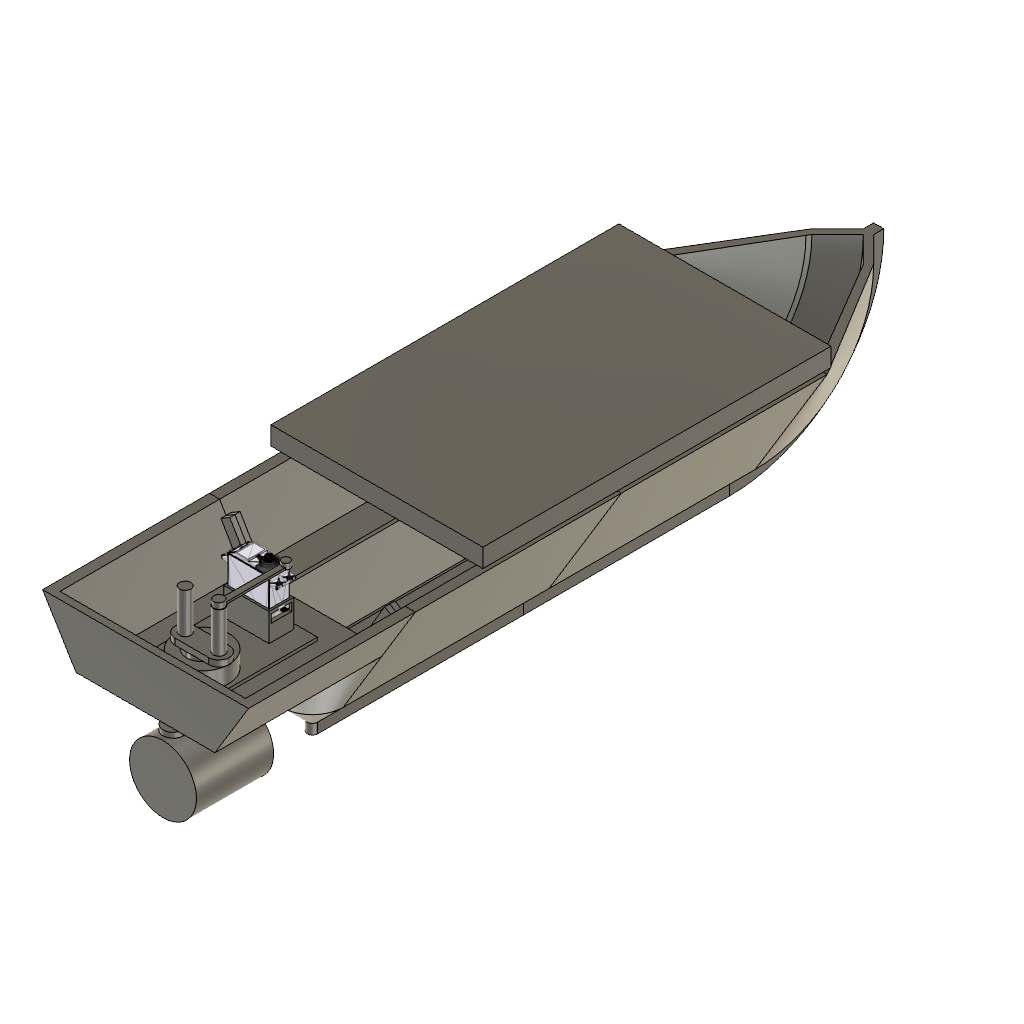
Aleph 0.2 (Autodesk Fusion 360 design; units mm, degrees)
part number: 2025-10-31-18-29-23-563
Autodesk Fusion 360 part; units mm, degrees
note: some values were not read from the file. Chosen so that the rebuilt part matches the saved one: a direction; which face or edge a step refers to. Set by a fixed rule: which sketch regions a step uses.
sketch "Skizze2" plane through (0, 0, 0) normal (0, 0, 1) x (1, 0, 0)
  line L0 (0, 0) -> (43, 0)
  line L1 (43, 0) -> (43, -97)
  line L2 (43, -97) -> (0, -97)
  line L3 (0, -97) -> (0, 0)
  dimension "d1" = 43
  dimension "d2" = 97
  constraint horizontal L0
  constraint vertical L1
  constraint horizontal L2
  constraint vertical L3
  constraint coincident L0.start L3.end
  measures "d1" distance of L0.start L0.end
  measures "d2" distance of L0.start L2.end
extrude "Extrusion1" add sketch "Skizze2" along normal blind 52 makes body 1
sketch "Skizze4" plane through (0, 0, 0) normal (0, 0, 1) x (1, 0, 0)
  line L0 (0, 0) -> (114.3, 0)
  line L1 (114.3, 0) -> (114.3, -187.452)
  line L2 (114.3, -187.452) -> (0, -187.452)
  line L3 (0, -187.452) -> (0, 0)
  dimension "d5" = 114.3
  dimension "d6" = 187.452
  constraint horizontal L0
  constraint vertical L1
  constraint horizontal L2
  constraint vertical L3
  constraint coincident L0.start L3.end
  measures "d5" distance of L0.start L0.end
  measures "d6" distance of L0.start L2.end
extrude "Extrusion2" add sketch "Skizze4" along normal blind 44.45 separate body makes body 2
move_body "Verschieben1" bodies 1 to x (0, -1, 0) y (1, 0, 0) z (0, 0, 1) at (47, -192, 0)
move_body "Verschieben2" bodies 2 to x (1, 0, 0) y (0, 1, 0) z (0, 0, 1) at (-60, 0, 0)
sketch "Skizze5" plane through (0, 0, 0) normal (0, 0, 1) x (1, 0, 0)
  line L0 (0, 0) -> (-57, 0)
  line L1 (-57, 0) -> (-57, 115)
  line L2 (-57, 115) -> (0, 115)
  line L3 (0, 115) -> (0, 0)
  dimension "d9" = 57
  dimension "d10" = 115
  constraint horizontal L0
  constraint vertical L1
  constraint horizontal L2
  constraint vertical L3
  constraint coincident L0.start L3.end
  measures "d9" distance of L0.start L0.end
  measures "d10" distance of L0.start L2.end
extrude "Extrusion3" add sketch "Skizze5" along normal blind 20 separate body makes body 3
move_body "Verschieben3" bodies 3 to x (-1, 0, 0) y (0, -1, 0) z (0, 0, 1) at (-32.12, -30.0306, 0.3149)
sketch "Skizze6" plane through (0, 0, 0) normal (0, 0, 1) x (1, 0, 0)
  line L0 (0, 0) -> (-340, 0)
  line L1 (-340, 0) -> (-340, 190)
  line L2 (-340, 190) -> (0, 190)
  line L3 (0, 190) -> (0, 0)
  dimension "d13" = 340
  dimension "d14" = 190
  constraint horizontal L0
  constraint vertical L1
  constraint horizontal L2
  constraint vertical L3
  constraint coincident L0.start L3.end
  measures "d13" distance of L0.start L0.end
  measures "d14" distance of L0.start L2.end
move_body "Verschieben5" bodies 1 to x (0, 1, 0) y (-1, 0, 0) z (0, 0, 1) at (-215.4447, -91.9643, -60)
sketch "Skizze8" plane through (0, 0, 19.9339) normal (0, 0, 1) x (-1, 0, 0)
  line L0 (-89.3962, 276.7581) -> (-89.3962, -63.2419)
  line L1 (-89.3962, -63.2419) -> (100.6038, -63.2419)
  line L2 (100.6038, -63.2419) -> (100.6038, 276.7581)
  line L3 (100.6038, 276.7581) -> (-89.3962, 276.7581)
  line L4 (0, 0) -> (206, 0)
  line L5 (206, 0) -> (206, -338)
  line L6 (206, -338) -> (0, -338)
  line L7 (0, -338) -> (0, 0)
  dimension "d17" = 206
  dimension "d18" = 338
  constraint horizontal L4
  constraint vertical L5
  constraint horizontal L6
  constraint vertical L7
  constraint coincident L4.start L7.end
  measures "d17" distance of L4.start L4.end
  measures "d18" distance of L4.start L6.end
extrude "Extrusion5" add sketch "Skizze8" along normal blind 18 separate body contours L1 L2 L4 L7 | L1 L2 L4 L5 L6 L7 makes body 4
move_body "Verschieben7" bodies 4 to x (1, 0, 0) y (0, 1, 0) z (0, 0, 1) at (95.4562, -274.0751, 0)
move_body "Verschieben8" bodies 4 to x (1, 0, 0) y (0, 1, 0) z (0, 0, 1) at (2.397, 0, -6.8914)
sketch "Skizze9" plane through (0, 0, 0) normal (0, 1, 0) x (1, 0, 0)
  line L0 (5, 140) -> (-5, 140)
  line L1 (-5, 140) -> (-30, 115)
  line L2 (29.8931, 115.1069) -> (5, 140)
  line L3 (-25, 110) -> (0, 135)
  line L4 (0, 135) -> (25, 110)
  line L5 (-25, 110) -> (-15, 110)
  line L6 (-15, 110) -> (-15, 106.5)
  line L7 (-15, 106.5) -> (-27.2273, 106.5)
  line L8 (5, 140) -> (5, 150)
  line L9 (5, 150) -> (-5, 150)
  line L10 (-5, 150) -> (-5, 140)
  line L11 (25, 110) -> (15, 110)
  line L12 (15, 110) -> (15, 106.5)
  line L13 (15, 106.5) -> (27.0682, 106.5)
  line L14 (-60.5574, 49.9522) -> (-35, 49.9522)
  line L15 (-35, 49.9522) -> (-35, 46.4522)
  line L16 (-35, 46.4522) -> (-62.6204, 46.4522)
  line L17 (60.4828, 49.9522) -> (35, 49.9522)
  line L18 (35, 49.9522) -> (35, 46.4522)
  line L19 (35, 46.4522) -> (62.551, 46.4522)
  line L20 (-90, 0) -> (-27.2273, 106.5)
  line L21 (-100, 0) -> (-30, 115)
  line L22 (90, 0) -> (27.0682, 106.5)
  line L23 (29.8931, 115.1069) -> (100, 0)
  line L24 (100, 0) -> (90, 0)
  line L25 (25, 110) -> (27.0682, 106.5)
  line L26 (-27.2273, 106.5) -> (-25, 110)
  line L27 (-100, 0) -> (-90, 0)
  line L28 (83.7574, 10.5643) -> (75.1482, 5.477)
  line L29 (75.1482, 5.477) -> (59.8863, 31.3048)
  line L30 (59.8863, 31.3048) -> (68.4956, 36.3921)
  line L31 (-68.5499, 36.3921) -> (-59.935, 31.3144)
  line L32 (-59.935, 31.3144) -> (-75.1683, 5.4697)
  line L33 (-75.1683, 5.4697) -> (-83.7832, 10.5474)
  line L34 (53.6547, 61.5074) -> (45.0455, 56.4201)
  line L35 (45.0455, 56.4201) -> (24.6963, 90.8572)
  line L36 (24.6963, 90.8572) -> (33.3055, 95.9445)
  line L37 (-33.4489, 95.9445) -> (-24.834, 90.8667)
  line L38 (-24.834, 90.8667) -> (-45.145, 56.4071)
  line L39 (-45.145, 56.4071) -> (-53.7599, 61.4849)
  line L40 (10, 125) -> (-10, 125)
  line L41 (71.7079, 46.4522) -> (-71.7247, 46.4522)
  line L42 (67.4445, 53.4522) -> (-67.4639, 53.4522)
  line L43 (0, 135) -> (0, 150)
  line L44 (90, 0) -> (-90, 0)
  dimension "d21" = 3.5
  dimension "d23" = 3.5
  dimension "d24" = 3.5
  dimension "d35" = 10
  dimension "d36" = 30
  dimension "d37" = 10
  dimension "d38" = 30
  dimension "d39" = 10
  dimension "d40" = 40
  dimension "d41" = 10
  dimension "d42" = 40
  constraint coincident L16.end L20
  constraint horizontal L16
  constraint coincident L14.start L20
  constraint horizontal L14
  constraint coincident L17.start L22
  constraint horizontal L17
  constraint coincident L19.end L22
  constraint horizontal L19
  constraint parallel L22 L25
  constraint horizontal L27
  constraint coincident L22 L28.start
  constraint perpendicular L22 L28
  constraint perpendicular L28 L29
  constraint coincident L22 L30.end
  constraint perpendicular L22 L30
  constraint coincident L20 L31.start
  constraint perpendicular L20 L31
  constraint perpendicular L31 L32
  constraint coincident L20 L33.end
  constraint perpendicular L20 L33
  constraint coincident L22 L34.start
  constraint perpendicular L22 L34
  constraint perpendicular L34 L35
  constraint coincident L22 L36.end
  constraint perpendicular L22 L36
  constraint coincident L20 L37.start
  constraint perpendicular L20 L37
  constraint perpendicular L37 L38
  constraint coincident L20 L39.end
  constraint perpendicular L20 L39
  constraint coincident L4 L40.start
  constraint coincident L3 L40.end
  constraint parallel L11 L40
  constraint coincident L23 L41.start
  constraint coincident L21 L41.end
  constraint parallel L19 L41
  constraint coincident L23 L42.start
  constraint coincident L21 L42.end
  constraint horizontal L42
  constraint midpoint L9 L43.end
  constraint perpendicular L9 L43
  constraint parallel L27 L44
  measures "d21" distance of L5.end L6.end
  measures "d23" distance of L11.end L12.end
  measures "d24" distance of L14.end L15.end
  measures "d35" distance of L28.start L28.end
  measures "d36" distance of L28.end L29.end
  measures "d37" distance of L31.start L31.end
  measures "d38" distance of L31.end L32.end
  measures "d39" distance of L34.start L34.end
  measures "d40" distance of L34.end L35.end
  measures "d41" distance of L37.end L37.start
  measures "d42" distance of L37.end L38.end
move_body "Verschieben9" bodies 2 to x (1, 0, 0) y (0, 1, 0) z (0, 0, 1) at (0, 0, 1.39)
move_body "Verschieben10" bodies 3 to x (1, 0, 0) y (0, 1, 0) z (0, 0, 1) at (0, 0, 5)
move_body "Verschieben11" bodies 1 to x (1, 0, 0) y (0, 1, 0) z (0, 0, 1) at (0, 0, 1.5638)
move_body "Verschieben12" bodies 4 to x (1, 0, 0) y (0, 1, 0) z (0, 0, 1) at (0, -63.155, 0.694)
sketch "Skizze11" plane through (0, 0, 0) normal (0, 1, 0) x (1, 0, 0)
  circle A0 centre (0, -70) radius 32.5
  dimension "d32" = 65
  measures "d32" diameter of A0
move_body "Verschieben16" bodies 4 to x (1, 0, 0) y (0, 1, 0) z (0, 0, 1) at (5.0085, 0, -7.0491)
extrude "Extrusion10" add sketch "Skizze9" against normal blind 200 separate body contours L0 L2 L4 L22 L23 L25 L42 L43 | L0 L1 L3 L20 L21 L26 L42 L43 | L22 L23 L41 L42 | L22 L23 L24 L41 | L20 L21 L41 L42 | L20 L21 L27 L41 makes body 5
move_body "Verschieben17" bodies 2 1 to x (1, 0, 0) y (0, 1, 0) z (0, 0, 1) at (0, -5, 0)
extrude "Extrusion11" add sketch "Skizze9" against normal blind 200 contours L5 L6 L7 L26 | L11 L12 L13 L25 | L17 L18 L19 L22 L41 | L14 L15 L16 L20 L41 bodies 5
extrude "Extrusion12" add sketch "Skizze9" against normal blind 200 contours L0 L8 L9 L43 | L0 L9 L10 L43 bodies 5
extrude "Extrusion13" add sketch "Skizze9" against normal blind 5 contours L3 L4 L40 | L22 L34 L35 L36 | L22 L28 L29 L30 | L20 L37 L38 L39 | L20 L31 L32 L33 bodies 5
extrude "Extrusion14" add sketch "Skizze9" along normal blind 5 from surface at -200 contours L3 L4 L40 | L22 L34 L35 L36 | L22 L28 L29 L30 | L20 L37 L38 L39 | L20 L31 L32 L33 bodies 5
revolve "Drehen2" add sketch "Skizze9" angle 90 about axis through (1.75, 0, 0) along (1, 0, 0) separate body contours L0 L2 L4 L22 L23 L25 L42 L43 | L0 L8 L9 L43 | L0 L1 L3 L20 L21 L26 L42 L43 | L0 L9 L10 L43 | L22 L23 L41 L42 | L22 L23 L24 L41 | L20 L21 L41 L42 | L20 L21 L27 L41 makes body 6
extrude "Extrusion15" add sketch "Skizze9" along normal blind 5 contours L3 L4 L40 | L22 L34 L35 L36 | L22 L28 L29 L30 | L20 L37 L38 L39 | L20 L31 L32 L33 bodies 6
copy_body "Körper kopieren/einfügen1" bodies 5 makes body 7
move_body "Verschieben18" bodies 7 to x (1, 0, 0) y (0, 1, 0) z (0, 0, 1) at (0, -200, 0)
sketch "Skizze12" plane through (0, 0, 0) normal (0, 0, 1) x (1, 0, 0)
  line L0 (-32.5, 0) -> (-32.5, -75)
  line L1 (-32.5, -75) -> (32.5, -75)
  line L2 (32.5, -75) -> (32.5, 0)
  line L3 (32.5, 0) -> (-32.5, 0)
  circle A0 centre (0, -17.2765) radius 1.15
  circle A1 centre (0, -37.2765) radius 1.15
  circle A2 centre (0, -57.2765) radius 1.15
  line L4 (3.25, -57.2765) -> (3.25, -17)
  line L5 (-3.25, -57.2765) -> (-3.25, -17.2765)
  arc A3 (3.25, -17) -> (-3.25, -17.2765) centre (0.0059, -17.2765) ccw
  arc A4 (-3.25, -57.2765) -> (3.25, -57.2765) centre (0, -57.2765) ccw
  dimension "d59" = 75
  dimension "d60" = 65
  dimension "d61" = 2.3
  dimension "d62" = 20
  dimension "d63" = 2.3
  dimension "d64" = 20
  dimension "d65" = 2.3
  constraint perpendicular L0 L1
  constraint perpendicular L1 L2
  constraint perpendicular L0 L3
  constraint vertical L4
  constraint vertical L5
  constraint tangent L5 A3
  constraint tangent L4 A4
  constraint tangent L5 A4
  measures "d59" distance of L0.start L0.end
  measures "d60" distance of L0.end L1.end
  measures "d61" diameter of A0
  measures "d62" distance of A0.centre A1.centre
  measures "d63" diameter of A1
  measures "d64" distance of A1.centre A2.centre
  measures "d65" diameter of A2
extrude "Extrusion16" add sketch "Skizze11" against normal blind 75 separate body makes body 8
extrude "Extrusion17" add sketch "Skizze12" along normal blind 4 from surface at 102.5 contours L4 L5 A3 A4 bodies 8
move_body "Verschieben19" bodies 8 to x (1, 0, 0) y (0, 1, 0) z (0, 0, 1) at (0, -436.8438, -182.9817)
other "Grundnetzelement1"
move_body "Verschieben20" bodies 8 to x (1, 0, 0) y (0, 1, 0) z (0, 0, 1) at (0, 0, 20)
other "Ändern1"
move_body "Verschieben21" bodies 8 to x (1, 0, 0) y (0, 1, 0) z (0, 0, 1) at (0, -25, 0)
other "Ändern2"
other "Netzreparatur1"
move_body "Verschieben22" bodies 8 to x (1, 0, 0) y (0, 1, 0) z (0, 0, 1) at (0, -30, 0)
other "Ändern3"
move_body "Verschieben23" bodies 8 to x (1, 0, 0) y (0, 1, 0) z (0, 0, 1) at (0, 31.8147, -24.8688)
other "Ändern4"
extrude "Extrusion18" add sketch "Skizze9" against normal blind 130 from surface at -400 separate body contours L22 L23 L41 L42 | L22 L23 L24 L41 | L14 L15 L17 L18 L20 L22 L41 L42 | L20 L21 L41 L42 | L17 L18 L19 L22 L41 | L20 L21 L27 L41 | L14 L15 L16 L20 L41 makes body 9
move_body "Verschieben24" bodies 8 to x (1, 0, 0) y (0, 1, 0) z (0, 0, 1) at (0, 20, 0)
extrude "Extrusion19" add sketch "Skizze9" against normal blind 5 from surface at -400 contours L22 L28 L29 L30 | L20 L31 L32 L33 bodies 9
revolve "Drehen3" add sketch "Skizze9" angle 180 about axis through (0, 0, 1.75) along (0, 0, 1) separate body contours L0 L1 L3 L20 L21 L26 L42 L43 | L0 L9 L10 L43 makes body 10
move_body "Verschieben25" bodies 10 to x (1, 0, 0) y (0, 1, 0) z (0, 0, 1) at (0, -400, 0)
combine "Kombinieren1" operation add target body 10 tool bodies 9
extrude "Extrusion20" add sketch "Skizze9" against normal blind 25 from surface at -530 contours L22 L23 L41 L42 | L22 L23 L24 L41 | L14 L15 L17 L18 L20 L22 L41 L42 | L20 L21 L41 L42 | L17 L18 L19 L22 L41 | L20 L21 L27 L41 | L14 L15 L16 L20 L41 bodies 10
move_body "Verschieben26" bodies 8 to x (1, 0, 0) y (0, 1, 0) z (0, 0, 1) at (0, -30, 0)
extrude "Extrusion21" add sketch "Skizze9" against normal blind 5 from surface at -400 contours L3 L4 L40 | L22 L34 L35 L36 | L20 L37 L38 L39 bodies 10
extrude "Extrusion22" add sketch "Skizze9" against normal blind 7 from surface at -555 contours L22 L23 L41 L42 | L22 L23 L24 L41 | L14 L15 L17 L18 L20 L22 L41 L42 | L20 L21 L41 L42 | L16 L19 L20 L22 L28 L29 L30 L31 L32 L33 L41 L44 | L17 L18 L19 L22 L41 | L20 L21 L27 L41 | L22 L28 L29 L30 | L14 L15 L16 L20 L41 | L20 L31 L32 L33 bodies 10
sketch "Skizze16" plane through (0, 0, 0) normal (0, 0, 1) x (1, 0, 0)
  circle A0 centre (0, -507) radius 10
  line L0 (0, -497) -> (-16.4, -497)
  line L1 (-16.4, -517) -> (0, -517)
  line L2 (16.4, -517) -> (0, -517)
  line L3 (16.4, -497) -> (0, -497)
  arc A1 (-16.4, -497) -> (-16.4, -517) centre (-16.4, -507) ccw
  arc A2 (16.4, -517) -> (16.4, -497) centre (16.4, -507) ccw
  circle A3 centre (16.4, -507) radius 5.5
  circle A4 centre (-16.4, -507) radius 5.5
  circle A5 centre (0, -507) radius 10.5
  dimension "d95" = 20
  dimension "d100" = 11
  dimension "d101" = 11
  dimension "d124" = 21
  constraint coincident A0 L0.start
  constraint coincident A0 L1.end
  constraint tangent A0 L1
  constraint parallel L0 L1
  constraint tangent A0 L2
  constraint tangent A0 L3
  constraint tangent L0 A1
  constraint tangent L3 A2
  constraint tangent L2 A2
  constraint concentric A2 A3
  constraint concentric A1 A4
  constraint concentric A0 A5
  measures "d95" diameter of A0
  measures "d100" diameter of A3
  measures "d101" diameter of A4
  measures "d124" diameter of A5
other "Ändern5"
other "Ändern6"
extrude "Extrusion23" add sketch "Skizze16" along normal blind 6 separate body contours A0 | A0 L2 L3 A5 | A0 L0 L1 A5 | L0 L1 A1 A5 | L2 L3 A2 A5 | A3 | A4 makes body 11
extrude "Extrusion24" add sketch "Skizze16" along normal blind 45 separate body contours A3 | A4 makes body 12 at (-11.7069, -509.8679, 30) makes body 13 at (20.7842, -503.6791, 30)
combine "Kombinieren2" operation add target body 13 tool bodies 11 12
move_body "Verschieben27" bodies 13 to x (1, 0, 0) y (0, 1, 0) z (0, 0, 1) at (0, 0, -40)
move_body "Verschieben28" bodies 13 to x (1, 0, 0) y (0, 1, 0) z (0, 0, 1) at (0, 0, -5)
extrude "Extrusion25" add sketch "Skizze16" against normal blind 30 from surface at -45 contours A0 bodies 13
sketch "Skizze17" plane through (0, 0, 0) normal (0, 0, 1) x (1, 0, 0)
  circle A0 centre (0, -507) radius 10
  circle A1 centre (0, -507) radius 15
  line L0 (9.9683, -518.2086) -> (9.9683, -535)
  line L1 (-10, -535) -> (-10, -518.1803)
  arc A2 (-10, -535) -> (9.9683, -535) centre (-0.0158, -535) ccw
  line L2 (10.0347, -495.8508) -> (10.0347, -479)
  line L3 (-10.0008, -495.8204) -> (-10.0008, -479)
  arc A3 (10.0347, -479) -> (-10.0008, -479) centre (0.017, -479) ccw
  line L4 (-10.0008, -495.8204) -> (-10, -518.1803)
  line L5 (9.9683, -518.2086) -> (10.0347, -495.8508)
  dimension "d109" = 30
  constraint concentric A0 A1
  constraint coincident A1 L0.start
  constraint vertical L0
  constraint coincident A1 L1.end
  constraint tangent L0 A2
  constraint tangent L1 A2
  constraint coincident A1 L2.start
  constraint vertical L2
  constraint coincident A1 L3.start
  constraint vertical L3
  constraint tangent L2 A3
  constraint tangent L3 A3
  measures "d109" diameter of A1
extrude "Extrusion26" add sketch "Skizze17" along normal blind 17.5 from surface at -75 separate body contours A0 A1 L4 L5 | A1 L5 | A0 A1 L4 L5 | A1 L4 makes body 14
extrude "Extrusion27" add sketch "Skizze17" against normal blind 5 from surface at -75 contours A0 | A0 A1 L4 L5 | A0 A1 L4 L5 | A1 L0 L1 A2 | A1 L2 L3 A3 bodies 14
sketch "Skizze18" plane through (0, 0, 0) normal (0, 0, 1) x (1, 0, 0)
  line L0 (100, 0) -> (-100, 0)
  line L1 (-100, 0) -> (-30, 115)
  line L2 (-30, 115) -> (-5, 140)
  line L3 (-5, 140) -> (-5, 150)
  line L4 (-5, 150) -> (5, 150)
  line L5 (5, 150) -> (5, 140)
  line L6 (5, 140) -> (30, 115)
  line L7 (30, 115) -> (100, 0)
  constraint horizontal L0
  constraint perpendicular L0 L3
  constraint perpendicular L3 L4
  constraint perpendicular L4 L5
sketch "Skizze19" plane through (0, 0, 0) normal (0, 0, 1) x (1, 0, 0)
  line L0 (100, -200) -> (-100, -200)
  line L1 (-100, -200) -> (-100, 0)
  line L2 (-100, 0) -> (100, 0)
  line L3 (100, 0) -> (100, -200)
  constraint horizontal L0
  constraint perpendicular L0 L1
  constraint perpendicular L1 L2
  constraint perpendicular L0 L3
sketch "Skizze20" plane through (0, 0, 0) normal (0, 0, 1) x (1, 0, 0)
  line L0 (100, -400) -> (-100, -400)
  line L1 (-100, -400) -> (-100, -200)
  line L2 (-100, -200) -> (100, -200)
  line L3 (100, -200) -> (100, -400)
  constraint horizontal L0
  constraint perpendicular L0 L1
  constraint perpendicular L1 L2
  constraint perpendicular L0 L3
sketch "Skizze21" plane through (0, 0, 0) normal (0, 0, 1) x (1, 0, 0)
  line L0 (100, -400) -> (-100, -400)
  line L1 (-100, -400) -> (-100, -562)
  line L2 (-100, -562) -> (100, -562)
  line L3 (100, -562) -> (100, -400)
  constraint horizontal L0
  constraint perpendicular L0 L1
  constraint perpendicular L1 L2
  constraint perpendicular L0 L3
extrude "Extrusion28" add sketch "Skizze21" along normal blind 6 separate body makes body 15
extrude "Extrusion29" add sketch "Skizze20" along normal blind 6 separate body makes body 16
extrude "Extrusion30" add sketch "Skizze19" along normal blind 6 separate body makes body 17
extrude "Extrusion31" add sketch "Skizze18" along normal blind 6 separate body makes body 18
move_body "Verschieben29" bodies 3 2 1 to x (1, 0, 0) y (0, 1, 0) z (0, 0, 1) at (0, 0, -40)
move_body "Verschieben30" bodies 3 2 1 to x (1, 0, 0) y (0, 1, 0) z (0, 0, 1) at (0, 0, -5)
extrude "Extrusion32" cut sketch "Skizze16" against normal blind 100 contours A0 | A0 L2 L3 A5 | A0 L0 L1 A5 | L0 L3 A5 | L1 L2 A5 bodies 10
sketch "Skizze22" plane through (0, 0, -46.4522) normal (0, 0, 1) x (-1, 0, 0)
  circle A0 centre (0, 507) radius 10.5
  line L0 (-62.551, 400) -> (62.6204, 400)
  line L1 (62.6204, 400) -> (62.6204, 555)
  line L2 (62.6204, 555) -> (-62.551, 555)
  line L3 (-62.551, 555) -> (-62.551, 400)
  line L4 (-30, 535) -> (40, 535)
  line L5 (40, 535) -> (40, 425)
  line L6 (40, 425) -> (-30, 425)
  line L7 (-30, 425) -> (-30, 535)
  line L8 (-10, 452) -> (30, 452)
  line L9 (30, 452) -> (30, 432)
  line L10 (30, 432) -> (-10, 432)
  line L11 (-10, 432) -> (-10, 452)
  line L12 (-12, 454) -> (32, 454)
  line L13 (32, 454) -> (32, 430)
  line L14 (32, 430) -> (-12, 430)
  line L15 (-12, 430) -> (-12, 454)
  line L16 (-10, 452) -> (-12, 452)
  line L17 (-10, 432) -> (-12, 432)
  constraint horizontal L4
  constraint vertical L5
  constraint horizontal L6
  constraint vertical L7
  constraint horizontal L8
  constraint vertical L9
  constraint horizontal L10
  constraint vertical L11
  constraint horizontal L12
  constraint vertical L13
  constraint horizontal L14
  constraint vertical L15
  constraint coincident L15 L16.end
  constraint perpendicular L15 L16
  constraint coincident L15 L17.end
  constraint perpendicular L15 L17
sketch "Skizze23" plane through (0, 0, -46.4522) normal (0, 0, 1) x (1, 0, 0)
  circle A0 centre (0, -507) radius 15
  circle A1 centre (0, -507) radius 26
  dimension "d127" = 30
  dimension "d128" = 52
  constraint concentric A0 A1
  measures "d127" diameter of A0
  measures "d128" diameter of A1
extrude "Extrusion33" add sketch "Skizze23" along normal blind 16 separate body makes body 19
extrude "Extrusion34" add sketch "Skizze22" along normal blind 3 separate body contours L4 L5 L6 L7 | L8 L9 L10 L12 L13 L14 L15 L16 L17 | L8 L9 L10 L11 | L11 L15 L16 L17 makes body 20
move_body "Verschieben31" bodies 19 to x (1, 0, 0) y (0, 1, 0) z (0, 0, 1) at (0, 0, 3)
other "Ändern7"
move_body "Verschieben32" bodies 13 14 to x (1, 0, 0) y (0, 1, 0) z (0, 0, 1) at (0, 0, -1.452)
move_body "Verschieben33" bodies 13 to x (1, 0, 0) y (0, 1, 0) z (0, 0, 1) at (0, 0, 19)
other "Ändern8"
extrude "Extrusion36" add sketch "Skizze22" along normal blind 19 contours L8 L9 L10 L12 L13 L14 L15 L16 L17 | L8 L9 L10 L11 | L11 L15 L16 L17 bodies 20
extrude "Extrusion37" add sketch "Skizze22" along normal blind 29 contours L8 L9 L10 L12 L13 L14 L15 L16 L17 | L11 L15 L16 L17 bodies 20
extrude "Extrusion38" add sketch "Skizze22" along normal blind 30 contours L8 L9 L10 L12 L13 L14 L15 L16 L17 | L11 L15 L16 L17 bodies 20
extrude "Extrusion39" cut sketch "Skizze22" along normal blind 8 from surface at 19 contours L11 L15 L16 L17 bodies 20
sketch "Skizze24" plane through (0, 0, 17.548) normal (0, 0, 1) x (-1, 0, 0)
  circle A0 centre (-16.3625, 507.0129) radius 3
  line L0 (-16.3625, 507.0129) -> (-16.3625, 442.0129)
  circle A1 centre (-16.3625, 442.0129) radius 2.5
  circle A2 centre (-16.3625, 507.0129) radius 5
  circle A3 centre (-16.3625, 442.0129) radius 4
  line L1 (-13.2385, 503.1089) -> (-13.5048, 444.8117)
  line L2 (-19.2283, 502.9156) -> (-18.9832, 445.0348)
  dimension "d145" = 6
  dimension "d146" = 65
  dimension "d147" = 5
  dimension "d148" = 10
  dimension "d149" = 8
  constraint coincident A0.centre L0.start
  constraint vertical L0
  constraint coincident L0.end A1.centre
  constraint concentric A0 A2
  constraint coincident A2 L1.start
  constraint coincident A3 L1.end
  constraint coincident A2 L2.start
  constraint coincident A3 L2.end
  measures "d145" diameter of A0
  measures "d146" distance of A0.centre L0.end
  measures "d147" diameter of A1
  measures "d148" diameter of A2
  measures "d149" diameter of A3
extrude "Extrusion41" add sketch "Skizze24" along normal blind 2 separate body makes body 21
extrude "Extrusion42" add sketch "Skizze24" along normal blind 4 contours A2 | A3 bodies 21
extrude "Extrusion43" add sketch "Skizze24" along normal blind 1.5 from surface at 4 contours A0 | A2 | A3 | A1 bodies 21
extrude "Extrusion9" [suppressed]
move_body "Verschieben13" [suppressed]
move_body "Verschieben14" [suppressed]
move_body "Verschieben15" [suppressed]
named bodies: "Battery", "JorgeBox", "Jorge", "EcoWorthySolarPanel", "DNYSYSJ Motor", "MiddleSection1", "FrontSection", "MiddleSection2", "DNYSYSJMotor", "AftSection", "ServoMechanism", "MotorAttachment", "AftSectionLid", "MiddleSection2Lid", "MiddleSection1Lid", "FrontSectionLid", "AxialBearing", "ServoPlatform", "ServoArms"
